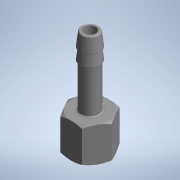
# Autodesk Inventor part: 2021 C-1/8-P-6
Saved by Autodesk Inventor 2021 (Build 250183000, 183)
## iProperties
Part Number: 2021 C-1/8-P-6
Material: Generic
Catalog Web Link: www.cadenas.de
Description: C-Barbed hose fitting
Vendor: FESTO
Document SubType Name: Modeling
Designer: partserver
Manufacturer: FESTO
Mass: 18 g
Surface Area: 21.755 cm^2
Volume: 1.77911 cm^3
Density: 1 g/cm^3
Appearance: PSOLRGB-175-175-175
Category: PARTsolutions
Company: FESTO
PSOL_IDENT_0: {$CADENAS_DATA\23d-libs\festo\parts\c\c\c.prj},163 {VTYP=3D},{NB=2021 C-1/8-P-6},{LINA=2021 C-1/8-P-
PSOL_IDENT_1: 6},{NN=C},{DATE=28.02.2020 14:10:26},{GEOMDATE=07.09.2015 09:33:02},{VERSION=},{LINEID=10},{WBVAR=},
PSOL_IDENT_2: {WBNUMERIC=}  {NB=2021 C-1/8-P-6},{LINA=2021 C-1/8-P-6},{KT=DUMMY},{TNR=2021},{TYP=C-1/8-P-6},{D1=G1
PSOL_IDENT_3: /8},{D2=7.000},{L1=36},{L2=24},{SW1=13},{CNSMASSEXACT=0.018},{D3=9.728},{D4=13.000},{D5=7.100},{D6=7
PSOL_IDENT_4: .000},{D7=8.500},{D8=6.000},{D9=4.000},{L3=12.000},{L4=2.500},{L5=33.000},{L6=4.000},{L7=5.000},{L8=
PSOL_IDENT_5: 2.500},{L9=1.500},{L10=26.500},{L11=4.000},{L12=5.000},{T1=9.000},{R1=3.500},{R2=0.400},{R3=0.200},{
PSOL_IDENT_6: R4=0.400},{W1=30.000},{W2=7.000}
NB: 2021 C-1/8-P-6
NN: C
NT: Barbed hose fitting
NBSYN: $TNR. $TYP.
LINA: 2021 C-1/8-P-6
CATALOG: Festo
TNR: 2021
TYP: C-1/8-P-6
D1: G1/8
D2: 7
L1: 36
L2: 24
SW1: 13
CNSMASSEXACT: 0.018
D3: 9.728
D4: 13
D5: 7.1
D6: 7
D7: 8.5
D8: 6
D9: 4
L3: 12
L4: 2.5
L5: 33
L6: 4
L7: 5
L8: 2.5
L9: 1.5
L10: 26.5
L11: 4
L12: 5
T1: 9
R1: 3.5
R2: 0.4
R3: 0.2
R4: 0.4
W1: 30
W2: 7
SUPPLIER: FESTO
ARTICLENO: 2021 C-1/8-P-6
BOMINFO: 2021 C-1/8-P-6
CREATOR: CADENAS GmbH
Title: 2021 C-1/8-P-6
Author: Cadenas PARTsolutions
Comments: Barbed hose fitting
Autodesk Inventor part; units mm, degrees
ref_plane "YZ Plane" through (0, 0, 0) normal (1, 0, 0) x (0, 1, 0)
ref_plane "XZ Plane" through (0, 0, 0) normal (0, 1, 0) x (-1, 0, 0)
ref_plane "XY Plane" through (0, 0, 0) normal (0, 0, 1) x (1, 0, 0)
sketch "Sketch_1" plane through (0, 0, 0) normal (1, 0, 0) x (0, 1, 0)
  line L0 (0, -12) -> (0, 0)
  line L1 (0, 0) -> (6.5, 0)
  line L2 (6.5, 0) -> (13, -3.7528)
  line L3 (13, -3.7528) -> (13, -8.2472)
  line L4 (13, -8.2472) -> (6.5, -12)
  line L5 (6.5, -12) -> (0, -12)
  line L6 (0, -12) -> (0, 0)
  constraints: 14 end point
revolve "Revolution1" add sketch "Sketch_1" angle 360 about axis through (0, 0, -12) along (0, 0, -1)
sketch "Sketch_2" plane through (0, 0, 0) normal (0, 0, 1) x (1, 0, 0)
  line L0 (-14, 14) -> (-14, -14)
  line L1 (-14, -14) -> (14, -14)
  line L2 (14, -14) -> (14, 14)
  line L3 (14, 14) -> (-14, 14)
  line L4 (-7.5056, 0) -> (-3.7528, -6.5)
  line L5 (-3.7528, -6.5) -> (3.7528, -6.5)
  line L6 (3.7528, -6.5) -> (7.5056, 0)
  line L7 (7.5056, 0) -> (3.7528, 6.5)
  line L8 (3.7528, 6.5) -> (-3.7528, 6.5)
  line L9 (-3.7528, 6.5) -> (-7.5056, 0)
  constraints: 20 end point
extrude "Extrusion1" cut sketch "Sketch_2" against normal blind 12
sketch "Sketch_3" plane through (0, 0, 0) normal (1, 0, 0) x (0, 1, 0)
  line L0 (0, -12) -> (0, 0)
  line L1 (0, 0) -> (4.864, 0)
  line L2 (4.864, 0) -> (4.283, -0.581)
  line L3 (4.283, -0.581) -> (4.283, -9.5)
  line L4 (4.283, -9.5) -> (3.55, -9.5)
  line L5 (3.55, -9.5) -> (3.55, -12)
  line L6 (3.55, -12) -> (0, -12)
  line L7 (0, -12) -> (0, 0)
  constraints: 16 end point
revolve "Revolution2" cut sketch "Sketch_3" angle 360 about axis through (0, 0, -12) along (0, 0, -1)
thread "Thread1" size "G9.728x0.907" designation "G 1/8" standard "ISO Pipe Threads" length 8.419
sketch "Sketch_4" plane through (0, 0, 0) normal (1, 0, 0) x (0, 1, 0)
  line L0 (0, -36) -> (0, -3)
  line L1 (2, -3) -> (2, -36)
  line L2 (2, -36) -> (2.5322, -36)
  arc A0 (2.5322, -36) -> (2.9292, -35.6487) centre (2.5322, -35.6) ccw
  line L3 (2.9292, -35.6487) -> (3.4725, -31.2244)
  arc A1 (3.4725, -31.2244) -> (3.2739, -31) centre (3.2739, -31.2) ccw
  line L4 (3.2739, -31) -> (3.0089, -31)
  line L5 (3.0089, -31) -> (3.4725, -27.2244)
  arc A2 (3.4725, -27.2244) -> (3.2739, -27) centre (3.2739, -27.2) ccw
  line L6 (3.2739, -27) -> (3, -27)
  line L7 (3, -27) -> (3, -12.4)
  arc A3 (3.4, -12) -> (3, -12.4) centre (3.4, -12.4) ccw
  line L8 (3.4, -12) -> (3.5, -12)
  line L9 (3.5, -12) -> (3.5, -9.5)
  line L10 (3.5, -9.5) -> (4.25, -9.5)
  line L11 (4.25, -9.5) -> (4.25, -7)
  line L12 (4.25, -7) -> (3.5, -7)
  line L13 (3.5, -7) -> (3.5, -5.5)
  arc A4 (3.5, -5.5) -> (2.4495, -3) centre (0, -5.5) ccw
  line L14 (2.4495, -3) -> (2, -3)
  constraints: 30 end point, 10 point on circle, 5 centre point
revolve "Revolution3" add sketch "Sketch_4" angle 360 about axis through (0, 0, -36) along (0, 0, -1)
body "Solid1"
